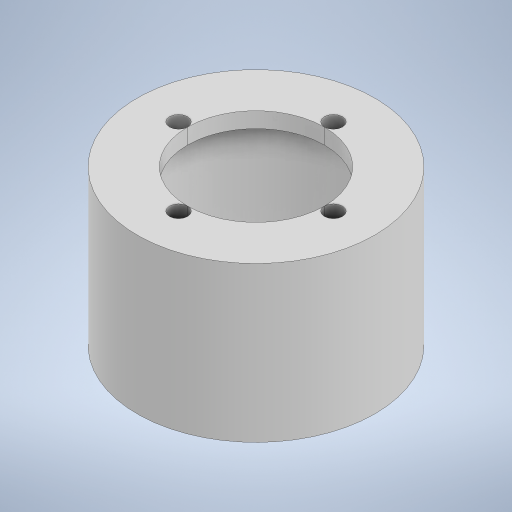
# Autodesk Inventor part: ColourSensor Scope
Saved by Autodesk Inventor 2024 (Build 280153020, 153B)
## iProperties
Created: 2024-01-08
Part Number: ColourSensor Scope
Material: Generic
Document SubType Name: Modeling
Designer: 2503645
Density: 1 g/cm^3
Appearance: Default
Author: 2503645
Autodesk Inventor part; units mm, degrees
ref_plane "YZ Plane" through (0, 0, 0) normal (1, 0, 0) x (0, 1, 0)
ref_plane "XZ Plane" through (0, 0, 0) normal (0, 1, 0) x (-1, 0, 0)
ref_plane "XY Plane" through (0, 0, 0) normal (0, 0, 1) x (1, 0, 0)
sketch "Sketch1" plane through (0, 0, 0) normal (0, 1, 0) x (-1, 0, 0)
  circle A0 centre (0, 0) radius 20
  circle A1 centre (0, 0) radius 15 construction
  circle A2 centre (0, -15) radius 1.75
  circle A3 centre (-15, 0) radius 1.75
  circle A4 centre (0, 15) radius 1.75
  circle A5 centre (15, 0) radius 1.75
  circle A6 centre (0, 0) radius 13.25
  point P0 (0, -13.25)
  point P1 (-13.25, 0)
  point P2 (0, 13.25)
  point P3 (13.25, 0)
  dimension "d0" = 40
  dimension "d1" = 30
  dimension "d2" = 3.5
  dimension "d3" = 3.5
  dimension "d4" = 3.5
  dimension "d5" = 3.5
  constraints: 7 centre point, 4 point on circle, 3 coincident, 1 tangent
  measures "d0" diameter of A0
  measures "d1" diameter of A1
  measures "d2" diameter of A2
  measures "d3" diameter of A3
  measures "d4" diameter of A4
  measures "d5" diameter of A5
extrude "Extrusion1" add sketch "Sketch1" along normal blind 3
sketch "Sketch2" plane through (0, 3, 0) normal (0, 1, 0) x (1, 0, 0)
  circle A0 centre (0, 0) radius 20
  circle A1 centre (0, 0) radius 23
  dimension "d8" = 46
  constraints: 2 centre point, 2 coincident
  measures "d8" diameter of A1
extrude "Extrusion2" add sketch "Sketch2" against normal blind 30
body "Solid1"
